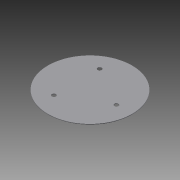
# Autodesk Inventor part: bottom
Saved by Autodesk Inventor 2015 SP1 (Build 190203100, 203)
## iProperties
Created: 2015-02-16
Part Number: bottom
Material: Wood (Birch)
Document SubType Name: Modeling
Designer: Jostein
Density: 0.55 g/cm^3
Appearance: Birch - Natural Polished
Author: Jostein
Autodesk Inventor part; units mm, degrees
ref_plane "YZ Plane" through (0, 0, 0) normal (1, 0, 0) x (0, 1, 0)
ref_plane "XZ Plane" through (0, 0, 0) normal (0, 1, 0) x (-1, 0, 0)
ref_plane "XY Plane" through (0, 0, 0) normal (0, 0, 1) x (1, 0, 0)
sketch "Sketch1" plane through (0, 0, 0) normal (0, 0, 1) x (1, 0, 0)
  circle A0 centre (0, 0) radius 245
  dimension "d0" = 490
  constraints: 1 centre point, 1 coincident
  measures "d0" diameter of A0
extrude "Extrusion1" add sketch "Sketch1" along normal blind 3
sketch "Sketch2" plane through (0, 0, 3) normal (0, 0, 1) x (1, 0, 0)
  point P0 (0, 0)
  point P1 (154, 0)
  point P2 (-77, 133.3679)
  point P3 (-77, -133.3679)
  dimension "d3" = 154
  dimension "d6" = 360
  constraints: 1 horizontal alignment, 4 other
  measures "d3" distance of point (0, 0) point (154, 0)
hole "Hole1" at (154, 0, 3) at (-77, 133.3679, 3) at (-77, -133.3679, 3) direction (0, 0, -1) diameter 24 end through all
body "Solid1"
